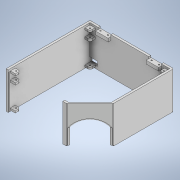
# Autodesk Inventor part: Box_Walls_2
Saved by Autodesk Inventor 2022 (Build 260153000, 153)
## iProperties
Created: 2023-02-27
Part Number: Box_Walls_2
Material: Generic
Document SubType Name: Modeling
Designer: zarek
Density: 1 g/cm^3
Appearance: Default
Author: zarek
Autodesk Inventor part; units mm, degrees
ref_plane "YZ Plane" through (0, 0, 0) normal (1, 0, 0) x (0, 1, 0)
sketch "Sketch1" plane through (0, 0, 0) normal (0, 1, 0) x (-1, 0, 0)
  line L0 (101.6, -101.6) -> (-101.6, -101.6)
  line L1 (-101.6, -101.6) -> (-101.6, 101.6)
  line L2 (-101.6, 101.6) -> (101.6, 101.6)
  line L3 (101.6, 101.6) -> (101.6, -101.6)
  line L4 (96.6, -96.6) -> (-96.6, -96.6)
  line L5 (-96.6, -96.6) -> (-96.6, 96.6)
  line L6 (-96.6, 96.6) -> (96.6, 96.6)
  line L7 (96.6, 96.6) -> (96.6, -96.6)
  line L8 (101.6, 101.6) -> (-40.4, 101.6)
  circle A0 centre (0, 0) radius 88.9
  circle A1 centre (0, 0) radius 109.3376
  line L9 (-40.4, 101.6) -> (-101.6, 40.4)
  line L10 (-45.4, 101.6) -> (-101.6, 45.4)
  line L11 (96.6, 96.6) -> (96.6, 101.6)
  line L12 (-45.4, 101.6) -> (-35.4, 101.6)
  line L13 (-35.4, 101.6) -> (-35.4, 96.6)
  line L14 (-35.4, 96.6) -> (-45.4, 96.6)
  line L15 (-45.4, 96.6) -> (-45.4, 101.6)
  point P0 (96.6, 51.2168)
  point P1 (101.6, 40.4)
  point P2 (101.6, -40.4)
  point P3 (96.6, -51.2168)
  point P4 (-96.6, 45.4)
  point P5 (-45.4, 96.6)
  dimension "d0" = 203.2
  dimension "d1" = 203.2
  dimension "d2" = 101.6
  dimension "d3" = 101.6
  dimension "d4" = 5
  dimension "d5" = 5
  dimension "d6" = 5
  dimension "d7" = 5
  dimension "d10" = 142
  dimension "d12" = 61.2
  dimension "d14" = 177.8
  dimension "d15" = 5
  dimension "d16" = 5
  dimension "d17" = 10
  constraints: 32 end point, 7 parallel, 6 point on line, 4 perpendicular, 3 horizontal, 2 centre point, 2 coincident, 2 point on circle
  measures "d0" distance between parallel lines of L2 L0
  measures "d1" distance between parallel lines of L1 L3
  measures "d2" distance from line of L0 point (0, 0)
  measures "d3" distance from line of L1 point (0, 0)
  measures "d4" distance between parallel lines of L4 L0
  measures "d5" distance between parallel lines of L1 L5
  measures "d6" distance between parallel lines of L2 L6
  measures "d7" distance between parallel lines of L3 L7
  measures "d10" distance of L2.end L8.end
  measures "d12" distance from line of L1 L8.end
  measures "d14" diameter of A0
  measures "d15" distance of L10.end L9.end
  measures "d16" distance of L10.start L8.end
  measures "d17" distance of L13.end L14.end
extrude "Extrusion1" add sketch "Sketch1" along normal blind 89.6 contours L0 A1 L4 L7 L3 | L0 A1 L4 | A1 L7 L3 | L0 L1 A1 L5 L4 | A1 L7 L11 L2 L3 | L1 L9 L5 A1 | L1 L10 A1 | A1 L10 L5 L9 | L5 L10 L6 L9 | L6 L9 L2 L13 | L15 A1 L9 | L6 L10 A1 L15 | A1 L15 L2 | A1 L10 L15
sketch "Sketch2" plane through (101.6, 0, 45.4) normal (0.7071068, 0, 0.7071068) x (0.7071068, 0, -0.7071068)
  line L0 (-179.888, 0) -> (-39.7394, 0) projected
  line L1 (-74.4788, 0) -> (-5, 0)
  line L2 (-5, 0) -> (-5, 38.1)
  line L3 (-5, 38.1) -> (-74.4788, 38.1)
  line L4 (-74.4788, 38.1) -> (-74.4788, 0)
  line L5 (0, 0) -> (0, 89.6) projected
  line L6 (-79.4788, 0) -> (-79.4788, 89.6) projected
  arc A0 (-5, 38.1) -> (-74.4788, 38.1) centre (-39.7394, 10.3696) ccw
  point P0 (-39.7394, 0)
  dimension "d20" = 5
  dimension "d21" = 5
  dimension "d22" = 38.1
  dimension "d33" = 44.45
  constraints: 8 end point, 2 parallel, 2 point on circle, 1 centre point, 1 horizontal, 1 perpendicular, 1 point on line
  measures "d20" distance between parallel lines of L5 L2
  measures "d21" distance between parallel lines of L4 L6
  measures "d22" distance between parallel lines of L0 L3
  measures "d33" radius of A0
extrude "Extrusion2" cut sketch "Sketch2" along normal mid plane 98.6
fillet "Fillet1" radius 3.175 2 edges at (101.6, 44.8, 45.4) (45.4, 44.8, 101.6)
sketch "Sketch4" plane through (101.6, 0, -101.6) normal (1, 0, 0) x (0, 0, -1)
  line L0 (-145.6849, 0) -> (-145.6849, 89.6) projected
  line L1 (-203.2, 0) -> (-203.2, 89.6) projected
  line L2 (-145.6849, 0) -> (-203.2, 0)
  line L3 (-203.2, 0) -> (-203.2, 2)
  line L4 (-203.2, 2) -> (-145.6849, 2)
  line L5 (-145.6849, 2) -> (-145.6849, 0)
  point P0 (-101.6, 0)
  point P1 (-203.2, 0)
  dimension "d28" = 2
  constraints: 8 end point, 2 parallel, 1 horizontal, 1 perpendicular, 1 point on line
  measures "d28" distance of L2.end L3.end
extrude "Extrusion3" cut sketch "Sketch4" against normal blind 57.658
fillet "Fillet3" radius 3.175 1 edges at (73.5, 54.8196, 73.5)
fillet "Fillet4" radius 3.175 4 edges at (48.9355, 40.5237, 98.0645) (48.9355, 20.05, 98.0645) (98.0645, 40.5237, 48.9355) (98.0645, 20.05, 48.9355)
sketch "Sketch5" plane through (-96.6, 0, -96.6) normal (0, 0, 1) x (1, 0, 0)
  line L0 (0, 0) -> (0, 89.6) projected
  line L1 (0, 0) -> (18.2, 0)
  line L2 (18.2, 0) -> (18.2, 17.8)
  line L3 (18.2, 17.8) -> (0, 17.8)
  line L4 (0, 17.8) -> (0, 0)
  line L5 (18.2, 0) -> (0, 0)
  line L6 (0, 0) -> (0, 7)
  line L7 (0, 7) -> (18.2, 7)
  line L8 (18.2, 7) -> (18.2, 0)
  point P0 (96.6, 0)
  point P1 (0, 7)
  point P2 (18.2, 7)
  point P3 (0, 17.8)
  dimension "d34" = 18.2
  dimension "d35" = 7
  dimension "d36" = 10.8
  constraints: 16 end point, 4 parallel, 2 horizontal, 2 perpendicular, 1 point on line
  measures "d34" distance of L3.end L2.end
  measures "d35" distance between parallel lines of L1 L7
  measures "d36" distance between parallel lines of L7 L3
extrude "Extrusion4" cut sketch "Sketch5" against normal blind 25.4 contours L0 L3 L2 L7
ref_plane "Work Plane3" through (-96.6, 7, -99.1) normal (0, 1, 0) x (1, 0, 0)
sketch "Sketch11" plane through (-96.6, 7, -99.1) normal (0, 1, 0) x (1, 0, 0)
  line L0 (0, -2.5) -> (0, -196.0064)
  line L1 (193.2, -2.5) -> (0, -2.5)
  line L2 (0, -2.5) -> (193.2, -2.5)
  line L3 (193.2, -144.8203) -> (141.8746, -196.0064)
  line L4 (193.2, -2.5) -> (193.2, -144.8203)
  line L5 (193.2, -144.8203) -> (141.8746, -196.0064)
  line L6 (141.8746, -196.0064) -> (0, -196.0064)
  line L7 (0, -196.0064) -> (0, -2.5)
  line L8 (0, -2.5) -> (7.0711, -9.5711)
  circle A0 centre (7.0711, -9.5711) radius 5.3203
  circle A1 centre (7.0711, -9.5711) radius 1
  line L9 (7.0711, -14.8914) -> (0, -14.8914)
  line L10 (7.0711, -9.5711) -> (7.0711, -14.8914)
  line L11 (7.0711, -9.5711) -> (12.3914, -9.5711)
  line L12 (12.3914, -2.5) -> (12.3914, -9.5711)
  line L13 (0, -196.0064) -> (7.0711, -188.9353)
  line L14 (0, -196.0064) -> (10, -196.0064) construction
  circle A2 centre (7.0711, -188.9353) radius 5
  circle A3 centre (7.0711, -188.9353) radius 1
  line L15 (7.0711, -188.9353) -> (12.0711, -188.9353)
  line L16 (12.0711, -196.0064) -> (12.0711, -188.9353)
  line L17 (7.0711, -188.9353) -> (7.0711, -183.9353)
  line L18 (0, -183.9353) -> (7.0711, -183.9353)
  line L19 (193.2, -2.5) -> (186.1289, -9.5711)
  circle A4 centre (186.1289, -9.5711) radius 5
  circle A5 centre (186.1289, -9.5711) radius 1
  line L20 (186.1289, -9.5711) -> (181.1289, -9.5711)
  line L21 (181.1289, -2.5) -> (181.1289, -9.5711)
  line L22 (186.1289, -9.5711) -> (186.1289, -14.5711)
  line L23 (193.2, -14.5711) -> (186.1289, -14.5711)
  line L24 (193.2, -142.5343) -> (193.2, -2.5)
  line L25 (0, -196.0064) -> (139.7178, -196.0064)
  line L26 (122, -124.8064) -> (198.2, -124.8064)
  line L27 (198.2, -188.3064) -> (198.2, 2.1936)
  line L28 (122, -124.8064) -> (122, -201.0064)
  line L29 (139.7178, -201.0064) -> (-5, -201.0064)
  line L30 (193.2, -124.8064) -> (183.2, -124.8064)
  circle A6 centre (183.2, -124.8064) radius 5
  circle A7 centre (183.2, -124.8064) radius 1
  line L31 (122, -196.0064) -> (122, -186.0064)
  line L32 (193.2, -2.5) -> (193.2, -144.5) projected
  line L33 (0, -2.5) -> (193.2, -2.5) projected
  line L34 (0, -200.7) -> (0, -2.5) projected
  line L35 (183.2, -119.8064) -> (193.2, -119.8064)
  line L36 (183.2, -124.8064) -> (183.2, -129.8064)
  line L37 (183.2, -129.8064) -> (193.2, -129.8064)
  point P0 (96.6, -99.1)
  point P1 (96.4746, -327.7)
  point P2 (-5, -201.0064)
  point P3 (0, -183.9353)
  point P4 (0, -196.0064)
  point P5 (12.3914, -2.5)
  point P6 (0, -14.8914)
  dimension "d96" = 10
  dimension "d97" = 2
  dimension "d98" = 10
  dimension "d99" = 45
  dimension "d100" = 10
  dimension "d101" = 2
  dimension "d102" = 10
  dimension "d103" = 10
  dimension "d104" = 2
  dimension "d105" = 76.2
  dimension "d106" = 76.2
  dimension "d109" = 2
  dimension "d113" = 228.6
  dimension "d114" = 0
  dimension "d115" = 0
  dimension "d116" = 0
  dimension "d117" = 0
  constraints: 68 end point, 15 point on line, 11 perpendicular, 8 centre point, 8 point on circle, 7 coincident, 5 horizontal, 3 parallel, 2 tangent, 2 vertical, 1 collinear, 1 equal length, 4 other
  measures "d96" distance of L0.start L8.end
  measures "d97" diameter of A1
  measures "d98" distance of L6.end L13.end
  measures "d99" angle of L14 L13
  measures "d100" diameter of A2
  measures "d101" diameter of A3
  measures "d102" distance of L1.start L19.end
  measures "d103" diameter of A4
  measures "d104" diameter of A5
  measures "d105" distance between parallel lines of L27 L28
  measures "d106" length of L26
  measures "d109" diameter of A7
  measures "d113" distance of point (96.475, -327.7) point (96.6, -99.1)
  measures "d114" distance between parallel lines of L32 L24
  measures "d115" distance between parallel lines of L33 L1
  measures "d116" distance between parallel lines of L34 L7
  measures "d117" distance between parallel lines of L6 L25
extrude "Extrusion8" add sketch "Sketch11" against normal blind 4.5 contours L8 A0 L9 L0 | L1 L12 A0 L8 | A0 L11 A1 L8 | L8 A1 L10 A0 | L18 A2 L13 L0 | L10 A1 L11 A0 | L1 L19 A4 L21 | L13 A2 L16 L6 | L17 A3 L13 A2 | A2 L15 A3 L17 | L4 L23 A4 L19 | L20 A5 L22 A4 | A4 L19 A5 L20 | L13 A3 L15 A2 | A4 L22 A5 L19 | L4 L26 A6 L35 | L4 L37 A6 L26 | A6 L26 A7 | A6 L36 A7 L26 | L26 A7 L36 A6
sketch "Sketch12" plane through (-101.6, 0, 101.6) normal (0, 0, 1) x (1, 0, 0)
  line L0 (0, 0) -> (5, 0) projected
  line L1 (5, 17.8) -> (5, 89.6) projected
  line L2 (0, 0) -> (5, 0)
  line L3 (5, 0) -> (5, 61.1)
  line L4 (5, 61.1) -> (0, 61.1)
  line L5 (0, 61.1) -> (0, 0)
  point P0 (101.6, 0)
  dimension "d120" = 61.1
  constraints: 8 end point, 2 parallel, 1 horizontal, 1 perpendicular, 1 point on line
  measures "d120" distance of L3.end L2.end
ref_plane "Work Plane4" through (-96.6, 61.1, 101.6) normal (0, 1, 0) x (-1, 0, 0)
sketch "Sketch13" plane through (-96.6, 61.1, 101.6) normal (0, 1, 0) x (-1, 0, 0)
  line L0 (0, -198.2) -> (0, -5)
  line L1 (-193.2, -198.2) -> (0, -198.2)
  line L2 (0, -198.2) -> (-193.2, -198.2)
  line L3 (-193.2, -56.1861) -> (-141.8746, -5)
  line L4 (-193.2, -198.2) -> (-193.2, -56.1861)
  line L5 (-193.2, -56.1861) -> (-141.8746, -5)
  line L6 (-141.8746, -5) -> (0, -5)
  line L7 (0, -5) -> (0, -198.2)
  line L8 (0, -198.2) -> (-7.0711, -191.1289)
  circle A0 centre (-7.0711, -191.1289) radius 5.3203
  circle A1 centre (-7.0711, -191.1289) radius 1
  line L9 (-7.0711, -185.8086) -> (0, -185.8086)
  line L10 (-7.0711, -191.1289) -> (-7.0711, -185.8086)
  line L11 (-7.0711, -191.1289) -> (-12.3914, -191.1289)
  line L12 (-12.3914, -198.2) -> (-12.3914, -191.1289)
  line L13 (0, -5) -> (-7.2124, -11.9268)
  line L14 (0, -5) -> (-9.998, -4.7981) construction
  circle A2 centre (-7.2124, -11.9268) radius 5
  circle A3 centre (-7.2124, -11.9268) radius 1
  line L15 (-7.2124, -11.9268) -> (-12.2124, -11.9073)
  line L16 (-12.1854, -5) -> (-12.2124, -11.9073)
  line L17 (-7.2124, -11.9268) -> (-7.2319, -16.9268)
  line L18 (0, -16.955) -> (-7.2319, -16.9268)
  line L19 (-193.2, -198.2) -> (-186.1289, -191.1289)
  circle A4 centre (-186.1289, -191.1289) radius 5
  circle A5 centre (-186.1289, -191.1289) radius 1
  line L20 (-186.1289, -191.1289) -> (-181.1289, -191.1289)
  line L21 (-181.1289, -198.2) -> (-181.1289, -191.1289)
  line L22 (-186.1289, -191.1289) -> (-186.1289, -186.1289)
  line L23 (-193.2, -186.1289) -> (-186.1289, -186.1289)
  line L24 (-193.2, -58.1657) -> (-193.2, -198.2)
  line L25 (0, -5) -> (-139.7178, -5)
  line L26 (-122, -76.2) -> (-198.2, -76.2)
  line L27 (-198.2, -12.5257) -> (-198.2, -203.0257)
  line L28 (-122, -76.2) -> (-122, 0)
  line L29 (-139.8151, 0) -> (4.9027, 0)
  line L30 (-193.2, -76.2) -> (-183.2973, -76.2)
  circle A6 centre (-183.2973, -76.2) radius 5
  circle A7 centre (-183.2973, -76.2) radius 1
  line L31 (-122, -5) -> (-122, -15)
  circle A8 centre (-122, -15) radius 5
  circle A9 centre (-122, -15) radius 1.75
  line L32 (-193.2, -198.2) -> (-193.2, -56.2)
  line L33 (0, -198.2) -> (-193.2, -198.2)
  line L34 (0, -0.1321) -> (0, -198.2)
  line L35 (-183.2973, -81.2) -> (-193.2, -81.2)
  line L36 (-183.2973, -76.2) -> (-183.2973, -71.2)
  line L37 (-183.2973, -71.2) -> (-193.2, -71.2)
  line L38 (-122, -15) -> (-127, -15)
  line L39 (-127, -15) -> (-127, -5)
  line L40 (-117, -15) -> (-117, -5)
  line L41 (0, 0) -> (0, -198.2) projected
  line L42 (0, -198.2) -> (-193.2, -198.2) projected
  line L43 (-198.2, -57.5151) -> (-198.2, -203.2) projected
  line L44 (0, -4.6936) -> (-12.0711, -4.6936) projected
  line L45 (5, 0) -> (0, 0) projected
  line L46 (-142, -5) -> (-132, -5) projected
  point P0 (-96.6, -101.6)
  point P1 (-96.6973, -101.7321)
  point P2 (-139.7178, -5)
  point P3 (-139.8151, 0)
  point P4 (4.9027, 0)
  point P5 (181.1289, -2.5)
  point P6 (193.2, -129.8064)
  point P7 (193.2, -119.8064)
  point P8 (117, -196.0064)
  point P9 (127, -196.0064)
  point P10 (0, -183.9353)
  point P11 (0, -196.0064)
  point P12 (12.3914, -2.5)
  point P13 (0, -14.8914)
  point P14 (-193.2, -71.2)
  point P15 (-193.2, -81.2)
  point P16 (0, -16.955)
  point P17 (0, -5)
  point P18 (-12.3914, -198.2)
  point P19 (0, -185.8086)
  dimension "d122" = 10
  dimension "d123" = 2
  dimension "d124" = 10
  dimension "d125" = 45
  dimension "d126" = 10
  dimension "d127" = 2
  dimension "d128" = 10
  dimension "d129" = 10
  dimension "d130" = 2
  dimension "d131" = 76.2
  dimension "d132" = 76.2
  dimension "d133" = 2
  dimension "d134" = 10
  dimension "d135" = 10
  dimension "d136" = 3.5
  dimension "d138" = 0
  dimension "d139" = 0
  dimension "d140" = 0
  dimension "d141" = 0
  dimension "d142" = 0
  dimension "d143" = 0
  dimension "d144" = 0
  dimension "d146" = 0
  dimension "d148" = 0
  constraints: 78 end point, 15 point on line, 12 perpendicular, 10 centre point, 10 point on circle, 9 coincident, 4 parallel, 3 tangent, 1 collinear, 1 equal length, 1 vertical, 10 other
  measures "d122" distance of L0.start L8.end
  measures "d123" diameter of A1
  measures "d124" distance of L6.end L13.end
  measures "d125" angle of L14 L13
  measures "d126" diameter of A2
  measures "d127" diameter of A3
  measures "d128" distance of L1.start L19.end
  measures "d129" diameter of A4
  measures "d130" diameter of A5
  measures "d131" distance between parallel lines of L27 L28
  measures "d132" length of L26
  measures "d133" diameter of A7
  measures "d134" distance of L31.start L31.end
  measures "d135" diameter of A8
  measures "d136" diameter of A9
  measures "d138" distance between parallel lines of L32 L24
  measures "d139" distance between parallel lines of L33 L1
  measures "d140" distance between parallel lines of L34 L7
  measures "d141" vertical extent of L6
  measures "d142" distance between parallel lines of L41 L7
  measures "d143" distance between parallel lines of L42 L1
  measures "d144" distance between parallel lines of L43 L27
  measures "d146" vertical extent of L45
  measures "d148" distance between parallel lines of L46 L6
extrude "Extrusion9" add sketch "Sketch13" along normal blind 5 contours L8 A0 L9 L0 | L1 L12 A0 L8 | A0 L11 A1 L8 | L8 A1 L10 A0 | L18 A2 L13 L0 | L10 A1 L11 A0 | L1 L19 A4 L21 | L13 A2 L16 L6 | L17 A3 L13 A2 | A2 L15 A3 L17 | L4 L23 A4 L19 | L20 A5 L22 A4 | A4 L19 A5 L20 | L13 A3 L15 A2 | A4 L22 A5 L19
sketch "Sketch14" plane through (-101.6, 0, 101.6) normal (0, 0, 1) x (1, 0, 0)
  line L0 (12.2319, 61.1) -> (5, 61.1) projected
  line L1 (5, 62) -> (5, 84.9)
  line L2 (5, 0) -> (5, 89.6) projected
  line L3 (5, 84.9) -> (137, 84.9)
  line L4 (137, 0) -> (137, 89.6) projected
  point P0 (101.6, 0)
  point P1 (5, 61.1)
  dimension "d151" = 22.9
  constraints: 4 end point, 2 point on line, 1 horizontal, 1 other
  measures "d151" distance of L1.start L1.end
ref_plane "Work Plane5" through (-96.6, 84.9, 101.6) normal (0, -1, 0) x (1, 0, 0)
sketch "Sketch15" plane through (-96.6, 84.9, 101.6) normal (0, -1, 0) x (1, 0, 0)
  line L0 (0, -198.2) -> (0, -5)
  line L1 (-193.2, -198.2) -> (0, -198.2)
  line L2 (0, -198.2) -> (-193.2, -198.2)
  line L3 (-193.2, -56.1861) -> (-141.8746, -5)
  line L4 (-193.2, -198.2) -> (-193.2, -56.1861)
  line L5 (-193.2, -56.1861) -> (-141.8746, -5)
  line L6 (-141.8746, -5) -> (0, -5)
  line L7 (0, -5) -> (0, -198.2)
  line L8 (0, -198.2) -> (-7.0711, -191.1289)
  circle A0 centre (-7.0711, -191.1289) radius 5.3203
  circle A1 centre (-7.0711, -191.1289) radius 1
  line L9 (-7.0711, -185.8086) -> (0, -185.8086)
  line L10 (-7.0711, -191.1289) -> (-7.0711, -185.8086)
  line L11 (-7.0711, -191.1289) -> (-12.3914, -191.1289)
  line L12 (-12.3914, -198.2) -> (-12.3914, -191.1289)
  line L13 (0, -5) -> (-7.2124, -11.9268)
  line L14 (0, -5) -> (-9.998, -4.7981) construction
  circle A2 centre (-7.2124, -11.9268) radius 5
  circle A3 centre (-7.2124, -11.9268) radius 1
  line L15 (-7.2124, -11.9268) -> (-12.2124, -11.9073)
  line L16 (-12.1854, -5) -> (-12.2124, -11.9073)
  line L17 (-7.2124, -11.9268) -> (-7.2319, -16.9268)
  line L18 (0, -16.955) -> (-7.2319, -16.9268)
  line L19 (-193.2, -198.2) -> (-186.1289, -191.1289)
  circle A4 centre (-186.1289, -191.1289) radius 5
  circle A5 centre (-186.1289, -191.1289) radius 1
  line L20 (-186.1289, -191.1289) -> (-181.1289, -191.1289)
  line L21 (-181.1289, -198.2) -> (-181.1289, -191.1289)
  line L22 (-186.1289, -191.1289) -> (-186.1289, -186.1289)
  line L23 (-193.2, -186.1289) -> (-186.1289, -186.1289)
  line L24 (-193.2, -58.1657) -> (-193.2, -198.2)
  line L25 (0, -5) -> (-139.7178, -5)
  line L26 (-122, -76.2) -> (-198.2, -76.2)
  line L27 (-198.2, -12.5257) -> (-198.2, -203.0257)
  line L28 (-122, -76.2) -> (-122, 0)
  line L29 (-139.8151, 0) -> (4.9027, 0)
  line L30 (-193.2, -76.2) -> (-183.2973, -76.2)
  circle A6 centre (-183.2973, -76.2) radius 5
  circle A7 centre (-183.2973, -76.2) radius 1
  line L31 (-122, -5) -> (-122, -15)
  circle A8 centre (-122, -15) radius 5
  circle A9 centre (-122, -15) radius 1.75
  line L32 (-193.2, -198.2) -> (-193.2, -56.2)
  line L33 (0, -198.2) -> (-193.2, -198.2)
  line L34 (0, -0.1321) -> (0, -198.2)
  line L35 (-183.2973, -81.2) -> (-193.2, -81.2)
  line L36 (-183.2973, -76.2) -> (-183.2973, -71.2)
  line L37 (-183.2973, -71.2) -> (-193.2, -71.2)
  line L38 (-122, -15) -> (-127, -15)
  line L39 (-127, -15) -> (-127, -5)
  line L40 (-117, -15) -> (-117, -5)
  line L41 (0, 0) -> (0, -198.2)
  line L42 (0, -198.2) -> (-193.2, -198.2)
  line L43 (-198.2, -57.5151) -> (-198.2, -203.2)
  line L44 (0, -4.6936) -> (-12.0711, -4.6936)
  line L45 (5, 0) -> (0, 0)
  line L46 (-142, -5) -> (-132, -5)
  line L47 (193.2, -198.2) -> (0, -198.2)
  line L48 (0, -198.2) -> (193.2, -198.2)
  line L49 (193.2, -56.1861) -> (141.8746, -5)
  line L50 (193.2, -198.2) -> (193.2, -56.1861)
  line L51 (193.2, -56.1861) -> (141.8746, -5)
  line L52 (141.8746, -5) -> (0, -5)
  line L53 (0, -198.2) -> (7.0711, -191.1289)
  circle A10 centre (7.0711, -191.1289) radius 5.3203
  circle A11 centre (7.0711, -191.1289) radius 1
  line L54 (7.0711, -185.8086) -> (0, -185.8086)
  line L55 (7.0711, -191.1289) -> (7.0711, -185.8086)
  line L56 (7.0711, -191.1289) -> (12.3914, -191.1289)
  line L57 (12.3914, -198.2) -> (12.3914, -191.1289)
  line L58 (0, -5) -> (7.2124, -11.9268)
  line L59 (0, -5) -> (9.998, -4.7981) construction
  circle A12 centre (7.2124, -11.9268) radius 5
  circle A13 centre (7.2124, -11.9268) radius 1
  line L60 (7.2124, -11.9268) -> (12.2124, -11.9073)
  line L61 (12.1854, -5) -> (12.2124, -11.9073)
  line L62 (7.2124, -11.9268) -> (7.2319, -16.9268)
  line L63 (0, -16.955) -> (7.2319, -16.9268)
  line L64 (193.2, -198.2) -> (186.1289, -191.1289)
  circle A14 centre (186.1289, -191.1289) radius 5
  circle A15 centre (186.1289, -191.1289) radius 1
  line L65 (186.1289, -191.1289) -> (181.1289, -191.1289)
  line L66 (181.1289, -198.2) -> (181.1289, -191.1289)
  line L67 (186.1289, -191.1289) -> (186.1289, -186.1289)
  line L68 (193.2, -186.1289) -> (186.1289, -186.1289)
  line L69 (193.2, -58.1657) -> (193.2, -198.2)
  line L70 (0, -5) -> (139.7178, -5)
  line L71 (122, -76.2) -> (198.2, -76.2)
  line L72 (198.2, -12.5257) -> (198.2, -203.0257)
  line L73 (122, -76.2) -> (122, 0)
  line L74 (139.8151, 0) -> (-4.9027, 0)
  line L75 (122, -5) -> (122, -15)
  circle A16 centre (122, -15) radius 5
  circle A17 centre (122, -15) radius 1.75
  line L76 (193.2, -198.2) -> (193.2, -56.2)
  line L77 (0, -198.2) -> (193.2, -198.2)
  line L78 (122, -15) -> (127, -15)
  line L79 (127, -15) -> (127, -5)
  line L80 (117, -15) -> (117, -5)
  line L81 (0, -198.2) -> (193.2, -198.2)
  line L82 (198.2, -57.5151) -> (198.2, -203.2)
  line L83 (0, -4.6936) -> (12.0711, -4.6936)
  line L84 (-5, 0) -> (0, 0)
  line L85 (142, -5) -> (132, -5)
  line L86 (193.2, -56.2) -> (142, -5) projected
  line L87 (142, -5) -> (193.2, -56.2)
  line L88 (142, -5) -> (142, -11.9268)
  line L89 (142, -11.9268) -> (186.2732, -56.2)
  line L90 (193.2, -57.5151) -> (193.2, -56.2) projected
  line L91 (186.2732, -56.2) -> (193.2, -56.2)
  circle A18 centre (165.7974, -32.3329) radius 1
  point P0 (96.6, -101.6)
  point P1 (-96.6, -101.6)
  point P2 (-96.6973, -101.7321)
  point P3 (-139.7178, -5)
  point P4 (-139.8151, 0)
  point P5 (4.9027, 0)
  point P6 (181.1289, -2.5)
  point P7 (193.2, -129.8064)
  point P8 (193.2, -119.8064)
  point P9 (117, -196.0064)
  point P10 (127, -196.0064)
  point P11 (0, -183.9353)
  point P12 (0, -196.0064)
  point P13 (12.3914, -2.5)
  point P14 (0, -14.8914)
  point P15 (-193.2, -71.2)
  point P16 (-193.2, -81.2)
  point P17 (0, -16.955)
  point P18 (0, -5)
  point P19 (-12.3914, -198.2)
  point P20 (0, -185.8086)
  point P21 (96.6, -101.6)
  point P22 (96.6973, -101.7321)
  point P23 (139.7178, -5)
  point P24 (139.8151, 0)
  point P25 (-4.9027, 0)
  point P26 (0, -16.955)
  point P27 (0, -185.8086)
  point P28 (12.3914, -198.2)
  point P29 (188.0675, -51.0675)
  point P30 (142, -5.1251)
  dimension "d153" = 10
  dimension "d154" = 2
  dimension "d155" = 10
  dimension "d156" = 45
  dimension "d157" = 10
  dimension "d158" = 2
  dimension "d159" = 10
  dimension "d160" = 10
  dimension "d161" = 2
  dimension "d162" = 76.2
  dimension "d163" = 76.2
  dimension "d164" = 2
  dimension "d165" = 10
  dimension "d166" = 10
  dimension "d167" = 3.5
  dimension "d168" = 0
  dimension "d169" = 0
  dimension "d170" = 0
  dimension "d171" = 0
  dimension "d172" = 0
  dimension "d173" = 0
  dimension "d174" = 0
  dimension "d175" = 0
  dimension "d176" = 0
  dimension "d179" = 0.3064
  dimension "d210" = 2
  dimension "d211" = 2.5
  constraints: 172 end point, 50 symmetric about line, 23 point on line, 19 centre point, 18 point on circle, 16 coincident, 13 perpendicular, 5 parallel, 3 tangent, 2 collinear, 2 vertical, 1 equal length, 28 other
  measures "d153" distance of L0.start L8.end
  measures "d154" diameter of A1
  measures "d155" distance of L6.end L13.end
  measures "d156" angle of L14 L13
  measures "d157" diameter of A2
  measures "d158" diameter of A3
  measures "d159" distance of L1.start L19.end
  measures "d160" diameter of A4
  measures "d161" diameter of A5
  measures "d162" distance between parallel lines of L27 L28
  measures "d163" length of L26
  measures "d164" diameter of A7
  measures "d165" distance of L31.start L31.end
  measures "d166" diameter of A8
  measures "d167" diameter of A9
  measures "d168" distance between parallel lines of L32 L24
  measures "d169" distance between parallel lines of L33 L1
  measures "d170" distance between parallel lines of L34 L7
  measures "d171" vertical extent of L6
  measures "d172" distance between parallel lines of L41 L7
  measures "d173" distance between parallel lines of L42 L1
  measures "d174" distance between parallel lines of L43 L27
  measures "d175" vertical extent of L45
  measures "d176" distance between parallel lines of L46 L6
  measures "d210" diameter of A18
  measures "d211" distance from line of L86 A18.centre
extrude "Extrusion10" add sketch "Sketch15" along normal blind 4.5 contours L53 A10 L57 L47 | L0 L54 A10 L53 | A10 L55 A11 L53 | L53 A11 L56 A10 | L0 L58 A12 L63 | A10 L56 A11 L55 | L66 A14 L64 L47 | L52 L61 A12 L58 | L62 A13 L60 A12 | A12 L58 A13 L62 | L64 A14 L68 L50 | L65 A15 L64 A14 | A14 L67 A15 L65 | A12 L60 A13 L58 | L64 A15 L67 A14 | L91 L89 L88 L49 L86 | L49 L88 L86
fillet "Fillet5" radius 3.175 2 edges at (101.6, 44.8, -101.6) (-101.6, 44.8, -101.6)
sketch "Sketch16" plane through (0, 89.6, 0) normal (0, 1, 0) x (1, 0, 0)
  line L0 (-96.6, -101.6) -> (-96.6, 96.6) projected
  line L1 (-96.6, -98.35) -> (-99.1, -98.35)
  line L2 (-99.1, -98.35) -> (-99.1, -100.1)
  line L3 (-99.1, -100.1) -> (-96.6, -100.1)
  line L4 (-96.6, -100.1) -> (-96.6, -98.35)
  line L5 (-101.6, -101.6) -> (-96.6, -101.6) projected
  line L6 (35.4, -96.6) -> (35.4, -101.6) projected
  line L7 (35.4, -100.1) -> (37.9, -100.1)
  line L8 (37.9, -100.1) -> (37.9, -98.35)
  line L9 (37.9, -98.35) -> (35.4, -98.35)
  line L10 (35.4, -98.35) -> (35.4, -100.1)
  line L11 (35.4, -101.6) -> (44.0849, -101.6) projected
  line L12 (45.4, -96.6) -> (35.4, -96.6) projected
  line L13 (-96.6, -100.1) -> (35.4, -100.1)
  line L14 (-101.6, 98.425) -> (-101.6, -101.6) projected
  point P0 (0, 0)
  dimension "d182" = 1.5
  dimension "d183" = 1.75
  dimension "d184" = 2.5
  dimension "d185" = 1.5
  dimension "d186" = 1.75
  dimension "d187" = 2.5
  dimension "d188" = 1.75
  dimension "d191" = 132
  dimension "d194" = 2.5
  constraints: 18 end point, 4 parallel, 2 horizontal, 2 perpendicular, 2 point on line
  measures "d182" distance between parallel lines of L5 L3
  measures "d183" distance between parallel lines of L3 L1
  measures "d184" distance between parallel lines of L0 L2
  measures "d185" distance between parallel lines of L11 L7
  measures "d186" distance between parallel lines of L7 L9
  measures "d187" distance between parallel lines of L6 L8
  measures "d188" distance between parallel lines of L9 L12
  measures "d191" distance of L3.end L7.start
  measures "d194" distance between parallel lines of L14 L2
extrude "Extrusion11" cut sketch "Sketch16" against normal through all
sketch "Sketch17" plane through (0, 0, 0) normal (0, -1, 0) x (1, 0, 0)
  point P0 (0, 0)
sketch "Sketch18" plane through (0, 89.6, 0) normal (0, 1, 0) x (1, 0, 0)
  line L0 (45.4, -96.6) -> (35.4, -96.6) projected
  line L1 (35.4, -101.6) -> (44.0849, -101.6) projected
  line L2 (35.4, -96.6) -> (39.0179, -96.6)
  line L3 (39.0179, -96.6) -> (39.0179, -101.6)
  line L4 (39.0179, -101.6) -> (35.4, -101.6)
  line L5 (35.4, -101.6) -> (35.4, -96.6)
  line L6 (-101.6, 98.425) -> (-101.6, -101.6) projected
  line L7 (-96.6, -101.6) -> (-96.6, -100.1) projected
  line L8 (-101.6, -96.6) -> (-96.6, -96.6)
  line L9 (-96.6, -96.6) -> (-96.6, -101.6)
  line L10 (-96.6, -101.6) -> (-101.6, -101.6)
  line L11 (-101.6, -101.6) -> (-101.6, -96.6)
  point P0 (0, 0)
  point P1 (-101.6, -101.6)
  constraints: 16 end point, 4 parallel, 3 point on line, 2 horizontal, 2 perpendicular
extrude "Extrusion12" add sketch "Sketch18" against normal blind 5
sketch "Sketch22" plane through (-96.6, 61.1, 101.6) normal (0, -1, 0) x (1, 0, 0)
  circle A0 centre (7.1759, -11.8979) radius 1.0267
  circle A1 centre (7.0845, -191.0815) radius 1.099
  circle A2 centre (186.1548, -191.1698) radius 1.0412
  point P0 (96.6, -101.6)
  constraints: 3 centre point
hole "Hole1" at (-89.4241, 61.1, 89.7021) at (-89.5155, 61.1, -89.4815) at (89.5548, 61.1, -89.5698) direction (0, 1, 0) diameter 2.85 depth 12.7 tip angle 118 countersink diameter 3 countersink angle 90 thread size "M3.5x0.6" class "6H" standard "ANSI Metric M Profile"
sketch "Sketch23" plane through (-96.6, 2.5, -99.1) normal (0, -1, 0) x (1, 0, 0)
  point P0 (96.6, 99.1)
sketch "Sketch24" plane through (-96.6, 2.5, -99.1) normal (0, -1, 0) x (1, 0, 0)
  circle A0 centre (7.0728, 188.9158) radius 1.0195
  circle A1 centre (7.0711, 9.5711) radius 1 projected
  circle A2 centre (7.0711, 9.5711) radius 1
  circle A3 centre (186.0543, 9.5711) radius 1.0028
  circle A4 centre (183.1847, 124.8098) radius 1.0762
  point P0 (96.6, 99.1)
  constraints: 4 centre point, 1 coincident
hole "Hole2" at (-89.5272, 2.5, 89.8158) at (-89.5289, 2.5, -89.5289) at (89.4543, 2.5, -89.5289) at (86.5847, 2.5, 25.7098) direction (0, 1, 0) diameter 2.85 depth 12.7 tip angle 118 countersink diameter 3 countersink angle 90 thread size "M3.5x0.6" class "6H" standard "ANSI Metric M Profile"
sketch "Sketch25" plane through (-96.6, 80.4, 101.6) normal (0, -1, 0) x (1, 0, 0)
  circle A0 centre (7.2045, -11.9025) radius 1.0659
  circle A1 centre (7.0584, -191.1632) radius 1.0343
  circle A2 centre (186.0543, -191.1289) radius 1.5 projected
  circle A3 centre (186.0543, -191.1289) radius 1.0077
  circle A4 centre (183.0986, -75.9599) radius 1.4972
  circle A5 centre (165.7974, -32.3329) radius 1 projected
  circle A6 centre (165.7974, -32.3329) radius 1
  point P0 (96.6, -101.6)
  constraints: 5 centre point, 2 coincident
hole "Hole3" at (69.1974, 80.4, 69.2671) at (86.4986, 80.4, 25.6401) at (89.4543, 80.4, -89.5289) at (-89.5416, 80.4, -89.5632) at (-89.3955, 80.4, 89.6975) direction (0, 1, 0) diameter 2.85 depth 12.7 tip angle 118 countersink diameter 5 countersink angle 90 thread size "M3.5x0.6" class "6H" standard "ANSI Metric M Profile"
sketch "Sketch26" plane through (0, 89.6, 0) normal (0, 1, 0) x (1, 0, 0)
  arc A0 (-98.425, 101.6) -> (-101.6, 98.425) centre (-98.425, 98.425) ccw projected
  line L0 (101.6, -44.0849) -> (101.6, 98.425) projected
  line L1 (98.425, 101.6) -> (-98.425, 101.6) projected
  line L2 (-46.1, 101.6) -> (-76.6, 101.6)
  line L3 (-96.6, 96.6) -> (96.6, 96.6) projected
  line L4 (-46.1, 96.6) -> (-76.6, 96.6)
  line L5 (-76.6, 101.6) -> (-76.6, 96.6)
  line L6 (-46.1, 101.6) -> (-46.1, 96.6)
  line L7 (-101.6, 98.425) -> (-101.6, -101.6) projected
  line L8 (0, 0) -> (0, 101.6)
  line L9 (46.1, 101.6) -> (76.6, 101.6)
  line L10 (46.1, 96.6) -> (76.6, 96.6)
  line L11 (76.6, 101.6) -> (76.6, 96.6)
  line L12 (46.1, 101.6) -> (46.1, 96.6)
  point P0 (98.425, 98.425)
  dimension "d220" = 30.5
  dimension "d221" = 25
  dimension "d224" = 5
  constraints: 18 end point, 5 symmetric about line, 3 point on line, 1 midpoint, 1 parallel, 1 perpendicular
  measures "d220" distance between parallel lines of L5 L6
  measures "d221" distance between parallel lines of L5 L7
  measures "d224" distance between parallel lines of L4 L2
extrude "Hinges Extrusion" cut sketch "Sketch26" against normal blind 4.2 contours L11 L3 L12 L1 | L6 L3 L5 L1
sketch "Sketch27" plane through (-96.6, 0, -96.6) normal (0, 0, 1) x (1, 0, 0)
  line L0 (50.5, 85.4) -> (20, 85.4) projected
  line L1 (20, 85.4) -> (50.5, 85.4)
  line L2 (50.5, 85.4) -> (50.5, 77.4)
  line L3 (50.5, 77.4) -> (20, 77.4)
  line L4 (20, 77.4) -> (20, 85.4)
  line L5 (173.2, 85.4) -> (142.7, 85.4) projected
  line L6 (173.2, 85.4) -> (142.7, 85.4)
  line L7 (142.7, 85.4) -> (142.7, 77.4)
  line L8 (142.7, 77.4) -> (173.2, 77.4)
  line L9 (173.2, 77.4) -> (173.2, 85.4)
  point P0 (96.6, 0)
  dimension "d225" = 8
  dimension "d226" = 8
  constraints: 16 end point, 4 parallel, 2 horizontal, 2 perpendicular
  measures "d225" distance of L1.end L2.end
  measures "d226" distance of L7.end L6.end
extrude "Extrusion14" add sketch "Sketch27" along normal blind 6.5
sketch "Sketch28" plane through (0, 85.4, 0) normal (0, 1, 0) x (1, 0, 0)
  line L0 (-76.6, 90.1) -> (-46.1, 90.1) projected
  line L1 (-46.1, 101.6) -> (-46.1, 96.6) projected
  line L2 (-76.6, 90.1) -> (-46.1, 90.1)
  line L3 (-46.1, 90.1) -> (-46.1, 101.6)
  line L4 (-46.1, 101.6) -> (-76.6, 101.6)
  line L5 (-76.6, 101.6) -> (-76.6, 90.1)
  line L6 (-76.6, 96.6) -> (-76.6, 90.1) projected
  line L7 (-76.6, 91.1) -> (-46.1, 91.1)
  line L8 (-62.066, 91.1) -> (-62.066, 96.35)
  line L9 (-62.066, 96.35) -> (-71.066, 96.35)
  line L10 (-62.066, 96.35) -> (-53.066, 96.35)
  circle A0 centre (-53.066, 96.35) radius 1
  circle A1 centre (-71.066, 96.35) radius 1
  line L11 (0, 0) -> (0, 101.6)
  line L12 (98.425, 101.6) -> (-98.425, 101.6) projected
  line L13 (76.6, 90.1) -> (46.1, 90.1)
  line L14 (46.1, 101.6) -> (46.1, 96.6)
  line L15 (76.6, 90.1) -> (46.1, 90.1)
  line L16 (46.1, 90.1) -> (46.1, 101.6)
  line L17 (46.1, 101.6) -> (76.6, 101.6)
  line L18 (76.6, 101.6) -> (76.6, 90.1)
  line L19 (76.6, 96.6) -> (76.6, 90.1)
  line L20 (76.6, 91.1) -> (46.1, 91.1)
  line L21 (62.066, 91.1) -> (62.066, 96.35)
  line L22 (62.066, 96.35) -> (71.066, 96.35)
  line L23 (62.066, 96.35) -> (53.066, 96.35)
  circle A2 centre (53.066, 96.35) radius 1
  circle A3 centre (71.066, 96.35) radius 1
  dimension "d229" = 1
  dimension "d230" = 5.25
  dimension "d231" = 9
  dimension "d232" = 9
  dimension "d233" = 2
  dimension "d234" = 2
  constraints: 40 end point, 15 symmetric about line, 6 point on line, 4 centre point, 4 coincident, 3 horizontal, 2 parallel, 2 perpendicular, 1 midpoint, 1 vertical, 2 other
  measures "d229" distance between parallel lines of L0 L7
  measures "d230" distance of L8.start L8.end
  measures "d231" distance of L8.end L9.end
  measures "d232" distance of L8.end L10.end
  measures "d233" diameter of A0
  measures "d234" diameter of A1
hole "Hole4" at (-71.066, 85.4, -96.35) at (-53.066, 85.4, -96.35) at (53.066, 85.4, -96.35) at (71.066, 85.4, -96.35) direction (0, -1, 0) diameter 2.85 depth 7 tip angle 118 countersink diameter 2.9 countersink angle 90 thread size "M3.5x0.6" class "6H" standard "ANSI Metric M Profile"
equation "\"d1\" = d0"
equation "\"d2\" = 0.5 * d0"
equation "\"d3\" = 0.5 * d0"
body "Solid1"
